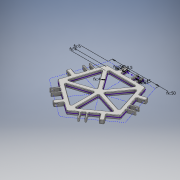
# Autodesk Inventor part: pentagon
Saved by Autodesk Inventor 2016 (Build 200138000, 138)
## iProperties
Created: 2016-11-12
Part Number: pentagon
Material: Generic
Document SubType Name: Modeling
Designer: Chris
Density: 1 g/cm^3
Appearance: Default
Author: Chris
Autodesk Inventor part; units mm, degrees
ref_plane "YZ Plane" through (0, 0, 0) normal (1, 0, 0) x (0, 1, 0)
ref_plane "XZ Plane" through (0, 0, 0) normal (0, 1, 0) x (-1, 0, 0)
ref_plane "XY Plane" through (0, 0, 0) normal (0, 0, 1) x (1, 0, 0)
sketch "Sketch1" plane through (0, 0, 0) normal (0, 0, 1) x (1, 0, 0)
  line L0 (25, 34.409548) -> (40.45085, -13.143278) construction
  line L1 (40.45085, -13.143278) -> (0, -42.53254) construction
  line L2 (0, -42.53254) -> (-40.45085, -13.143278) construction
  line L3 (-40.45085, -13.143278) -> (-25, 34.409548) construction
  line L4 (-25, 34.409548) -> (25, 34.409548) construction
  line L5 (20.640745, 28.409548) -> (33.397427, -10.851482)
  line L6 (33.397427, -10.851482) -> (0, -35.116133)
  line L7 (0, -35.116133) -> (-33.397427, -10.851482)
  line L8 (-33.397427, -10.851482) -> (-20.640745, 28.409548)
  line L9 (-20.640745, 28.409548) -> (20.640745, 28.409548)
  line L10 (0, -35.116133) -> (0, 0) construction
  line L11 (-17.734575, 24.409548) -> (-28.695145, -9.323618)
  line L12 (-28.695145, -9.323618) -> (0, -30.171861)
  line L13 (0, -30.171861) -> (28.695145, -9.323618)
  line L14 (28.695145, -9.323618) -> (17.734575, 24.409548)
  line L15 (17.734575, 24.409548) -> (-17.734575, 24.409548)
  line L16 (-7.5, 34.409548) -> (7.5, 34.409548) construction
  line L17 (4, 34.409548) -> (5.5, 34.409548) construction
  line L18 (5.5, 34.409548) -> (9.5, 34.409548) construction
  line L19 (11, 34.409548) -> (9.5, 34.409548) construction
  line L20 (-9.5, 34.409548) -> (-5.5, 34.409548) construction
  line L21 (-9.5, 28.409548) -> (-5.5, 28.409548)
  line L22 (-5.5, 28.409548) -> (-5.5, 36.409548)
  line L23 (-5.5, 36.409548) -> (-9.5, 36.409548)
  line L24 (-9.5, 36.409548) -> (-9.5, 28.409548)
  line L25 (4, 36.409548) -> (5.5, 36.409548)
  line L26 (5.5, 36.409548) -> (5.5, 28.409548)
  line L27 (5.5, 28.409548) -> (4, 28.409548)
  line L28 (4, 28.409548) -> (4, 36.409548)
  line L29 (9.5, 36.409548) -> (11, 36.409548)
  line L30 (11, 36.409548) -> (11, 28.409548)
  line L31 (11, 28.409548) -> (9.5, 28.409548)
  line L32 (9.5, 28.409548) -> (9.5, 36.409548)
  line L33 (-9.5, 34.409548) -> (-9, 34.409548)
  line L34 (-9.5, 34.409548) -> (-9.5, 35.909548)
  line L35 (-6, 34.409548) -> (-5.5, 34.409548)
  line L36 (-5.5, 34.409548) -> (-5.5, 35.909548)
  arc A0 (-9, 34.409548) -> (-9.5, 35.909548) centre (-11.5, 34.409548) ccw
  arc A1 (-5.5, 35.909548) -> (-6, 34.409548) centre (-3.5, 34.409548) ccw
  line L37 (5.5, 35.909548) -> (5.5, 34.409548)
  line L38 (5.5, 34.409548) -> (6, 34.409548)
  line L39 (9.5, 35.909548) -> (9.5, 34.409548)
  line L40 (9.5, 34.409548) -> (9, 34.409548)
  arc A2 (6, 34.409548) -> (5.5, 35.909548) centre (3.5, 34.409548) ccw
  arc A3 (9.5, 35.909548) -> (9, 34.409548) centre (11.5, 34.409548) ccw
  line L41 (-17.734575, 24.409548) -> (0, 0) construction
  line L42 (-28.695145, -9.323618) -> (0, 0) construction
  line L43 (17.734575, 24.409548) -> (0, 0) construction
  line L44 (28.695145, -9.323618) -> (0, 0) construction
  line L45 (0, 0) -> (-23.21486, 7.542965) construction
  line L46 (0, 24.409548) -> (0, 0) construction
  line L47 (0, 0) -> (23.21486, 7.542965) construction
  line L48 (0, 0) -> (14.347572, -19.747739) construction
  line L49 (-14.347572, -19.747739) -> (0, 0) construction
  line L50 (-18.498507, 22.058407) -> (-3.236068, 1.051462)
  line L51 (-3.236068, 1.051462) -> (-27.931213, -6.972477)
  line L52 (-15.262439, 24.409548) -> (0, 3.402603)
  line L53 (15.262439, 24.409548) -> (0, 3.402603)
  line L54 (18.498507, 22.058407) -> (3.236068, 1.051462)
  line L55 (27.931213, -6.972477) -> (3.236068, 1.051462)
  line L56 (26.695145, -10.776703) -> (2, -2.752764)
  line L57 (2, -2.752764) -> (2, -28.718776)
  line L58 (-2, -28.718776) -> (-2, -2.752764)
  line L59 (-2, -2.752764) -> (-26.695145, -10.776703)
  point P0 (0, 34.409548)
  dimension "d0" = 50
  dimension "d1" = 6
  dimension "d2" = 4
  dimension "d3" = 15
  dimension "d4" = 1.5
  dimension "d5" = 4
  dimension "d6" = 4
  dimension "d9" = 4
  dimension "d12" = 3
  dimension "d13" = 0.5
  dimension "d26" = 4
  constraints: 120 end point, 33 point on line, 16 parallel, 10 equal length, 9 midpoint, 8 horizontal, 8 point on circle, 7 coincident, 6 perpendicular, 5 vertical, 4 centre point, 2 collinear, 2 equal radius, 19 other
  measures "d0" distance of L3.end L0.start
  measures "d1" distance between parallel lines of L9 L4
  measures "d2" distance between parallel lines of L9 L15
  measures "d3" distance of L16.start L16.end
  measures "d4" distance of L19.start L18.end
  measures "d5" distance of L17.end L18.end
  measures "d6" distance of L20.start L20.end
  measures "d9" diameter of L23 L4
  measures "d12" diameter of L34.end L33
  measures "d13" distance of L20.start L33.end
  measures "d26" distance between parallel lines of L52 L50
extrude "Extrusion3" add sketch "Sketch1" along normal mid plane 4 contours L5 L6 L7 L8 L9 | L15 L52 L53 L14 L54 L55 L13 L56 L57 L12 L58 L59 L11 L51 L50
extrude "Extrusion2" add sketch "Sketch1" along normal mid plane 4 contours L9 L32 L29 L30 | L9 L28 L25 L26 | L24 L33 A0 L23 L22 A1 L35 L9 | L24 A0 L33 | L35 A1 L22
revolve "Revolution1" add sketch "Sketch1" angle 360 about axis through (-25, 34.409548, 0) along (1, 0, 0) contours L40 A3 L32 | L26 A2 L38
revolve "Revolution3" cut sketch "Sketch1" angle 360 about axis through (-9.5, 34.409548, 0) along (1, 0, 0) contours L24 A0 L33 | L35 A1 L22
fillet "Fillet5" radius 1 20 edges at (-20.6407, 28.4095, 0) (20.6407, 28.4095, 0) (33.3974, -10.8515, 0) (0, -35.1161, 0) (-33.3974, -10.8515, 0) (-18.4985, 22.0584, 0) (-15.2624, 24.4095, 0) (15.2624, 24.4095, 0) (0, 3.4026, 0) (-3.2361, 1.0515, 0) (-2, -2.7528, 0) (2, -2.7528, 0) (3.2361, 1.0515, 0) (-27.9312, -6.9725, 0) (-26.6951, -10.7767, 0) (-2, -28.7188, 0) (2, -28.7188, 0) (26.6951, -10.7767, 0) (27.9312, -6.9725, 0) (18.4985, 22.0584, 0)
pattern_circular "Circular Pattern1" count 5 over 360 about axis through (0, 0, -10) along (0, 0, 1) of "Extrusion2", "Revolution1", "Revolution3"
fillet "Fillet4" radius 0.75 60 edges at (-30.3002, -22.9903, 0) (-29.0867, -23.872, 0) (-25.8506, -26.2231, 0) (-24.6371, -27.1048, 0) (-16.9514, -32.6888, 0) (-13.7153, -35.0399, 0) (29.0867, -23.872, 0) (25.8506, -26.2231, 0) (18.1649, -31.8071, 0) (16.9514, -32.6888, 0) (13.7153, -35.0399, 0) (12.5018, -35.9216, 0) (38.0267, 0.7895, 0) (37.5632, 2.2161, 0) (36.3271, 6.0204, 0) (35.8636, 7.4469, 0) (32.9279, 16.482, 0) (31.6919, 20.2862, 0) (-9.5, 36.4095, 0) (-5.5, 36.4095, 0) (4, 36.4095, 0) (5.5, 36.4095, 0) (9.5, 36.4095, 0) (11, 36.4095, 0) (-31.6919, 20.2862, 0) (-31.2284, 21.7128, 0) (-32.9279, 16.482, 0) (-33.3915, 15.0554, 0) (-36.3271, 6.0204, 0) (-37.5632, 2.2161, 0) (-9.5, 28.4095, 0) (-5.5, 28.4095, 0) (4, 28.4095, 0) (5.5, 28.4095, 0) (9.5, 28.4095, 0) (11, 28.4095, 0) (24.0834, 17.8141, 0) (25.3195, 14.0098, 0) (28.2552, 4.9748, 0) (28.7187, 3.5482, 0) (29.9547, -0.256, 0) (30.4183, -1.6826, 0) (24.3844, -17.3998, 0) (21.1483, -19.751, 0) (13.4626, -25.3349, 0) (12.2491, -26.2166, 0) (9.0131, -28.5678, 0) (7.7995, -29.4494, 0) (-9.0131, -28.5678, 0) (-12.2491, -26.2166, 0) (-21.1483, -19.751, 0) (-19.9348, -20.6327, 0) (-25.5979, -16.5182, 0) (-24.3844, -17.3998, 0) (-29.9547, -0.256, 0) (-28.7187, 3.5482, 0) (-25.783, 12.5833, 0) (-25.3195, 14.0098, 0) (-24.0834, 17.8141, 0) (-23.6199, 19.2407, 0)
chamfer "Chamfer2" distance 0.4 angle 45 244 edges at (-15.0821, 28.4095, 2) (-20.502, 28.2186, 2) (-22.1267, 23.8363, 2) (-23.7609, 19.5175, 2) (-27.4241, 20.4767, 2) (-31.4151, 20.4272, 2) (-31.0873, 21.436, 2) (-27.8877, 19.0501, 2) (-24.3602, 17.673, 2) (-24.7015, 15.912, 2) (-25.4605, 14.2866, 2) (-29.1237, 15.2459, 2) (-32.7869, 16.2052, 2) (-33.1147, 15.1964, 2) (-29.5872, 13.8193, 2) (-26.0598, 12.4422, 2) (-27.2508, 8.0657, 2) (-28.8597, 3.825, 2) (-32.5229, 4.7843, 2) (-36.1861, 5.7436, 2) (-36.9452, 4.1182, 2) (-37.2864, 2.3572, 2) (-33.759, 0.9801, 2) (-30.2315, -0.397, 2) (-31.6797, -5.5649, 2) (-33.1729, -10.7785, 2) (-29.5072, -13.6779, 2) (-25.9047, -16.5668, 2) (-27.949, -19.7542, 2) (-29.1353, -23.5651, 2) (-29.9933, -22.9417, 2) (-26.7355, -20.6359, 2) (-24.3358, -17.7067, 2) (-22.7663, -18.5754, 2) (-21.4551, -19.7996, 2) (-23.4994, -22.9871, 2) (-24.6857, -26.798, 2) (-25.5438, -26.1745, 2) (-22.2859, -23.8687, 2) (-19.8862, -20.9395, 2) (-16.092, -23.4246, 2) (-12.556, -26.2652, 2) (-14.6003, -29.4527, 2) (-16.6446, -32.6402, 2) (-15.3334, -33.8643, 2) (-13.7639, -34.7331, 2) (-11.3642, -31.8038, 2) (-8.9645, -28.8746, 2) (-4.497, -31.8488, 2) (0, -34.8801, 2) (3.8903, -32.2897, 2) (7.7509, -29.7563, 2) (10.1507, -32.6855, 2) (13.4085, -34.9913, 2) (12.5504, -35.6147, 2) (11.3642, -31.8038, 2) (9.3199, -28.6164, 2) (10.6311, -27.3922, 2) (12.2005, -26.5235, 2) (14.6003, -29.4527, 2) (17.8581, -31.7585, 2) (17, -32.3819, 2) (15.8138, -28.571, 2) (13.7695, -25.3835, 2) (17.3055, -22.543, 2) (21.0997, -20.0578, 2) (23.4994, -22.9871, 2) (25.8992, -25.9163, 2) (27.4686, -25.0476, 2) (28.7798, -23.8234, 2) (26.7355, -20.6359, 2) (24.6912, -17.4484, 2) (28.9004, -14.1188, 2) (33.1729, -10.7785, 2) (31.9115, -6.2782, 2) (30.6951, -1.8236, 2) (34.2225, -0.4465, 2) (37.4222, 1.9393, 2) (37.7499, 0.9306, 2) (33.759, 0.9801, 2) (30.0958, 0.0208, 2) (29.3367, 1.6461, 2) (28.9955, 3.4072, 2) (32.5229, 4.7843, 2) (35.7226, 7.1701, 2) (36.0503, 6.1614, 2) (32.0594, 6.2109, 2) (28.3962, 5.2516, 2) (26.7873, 9.4923, 2) (25.5963, 13.8688, 2) (29.1237, 15.2459, 2) (32.6511, 16.623, 2) (-15.0821, 28.4095, -2) (-9.7197, 28.6292, -2) (-9.5, 32.4095, -2) (-9.2803, 36.1899, -2) (-7.5, 36.4095, -2) (-5.7197, 36.1899, -2) (-5.5, 32.4095, -2) (-5.2803, 28.6292, -2) (-0.75, 28.4095, -2) (3.7803, 28.6292, -2) (4, 32.4095, -2) (4.2197, 36.1899, -2) (5.2803, 36.1899, -2) (5.5, 32.4095, -2) (5.7197, 28.6292, -2) (7.5, 28.4095, -2) (9.2803, 28.6292, -2) (9.5, 32.4095, -2) (9.7197, 36.1899, -2) (10.7803, 36.1899, -2) (11, 32.4095, -2) (11.2197, 28.6292, -2) (15.8321, 28.4095, -2) (20.502, 28.2186, -2) (22.3585, 23.123, -2) (24.2245, 18.0909, -2) (27.8877, 19.0501, -2) (31.5508, 20.0094, -2) (32.3099, 18.3841, -2) (32.6511, 16.623, -2) (29.1237, 15.2459, -2) (25.5963, 13.8688, -2) (26.7873, 9.4923, -2) (28.3962, 5.2516, -2) (32.0594, 6.2109, -2) (35.7226, 7.1701, -2) (36.0503, 6.1614, -2) (32.5229, 4.7843, -2) (28.9955, 3.4072, -2) (29.3367, 1.6461, -2) (30.0958, 0.0208, -2) (33.759, 0.9801, -2) (37.4222, 1.9393, -2) (37.7499, 0.9306, -2) (34.2225, -0.4465, -2) (30.6951, -1.8236, -2) (31.9115, -6.2782, -2) (33.1729, -10.7785, -2) (28.9004, -14.1188, -2) (24.6912, -17.4484, -2) (26.7355, -20.6359, -2) (28.7798, -23.8234, -2) (27.4686, -25.0476, -2) (25.8992, -25.9163, -2) (23.4994, -22.9871, -2) (21.0997, -20.0578, -2) (17.3055, -22.543, -2) (13.7695, -25.3835, -2) (15.8138, -28.571, -2) (17.8581, -31.7585, -2) (17, -32.3819, -2) (14.6003, -29.4527, -2) (12.2005, -26.5235, -2) (10.6311, -27.3922, -2) (9.3199, -28.6164, -2) (11.3642, -31.8038, -2) (13.4085, -34.9913, -2) (12.5504, -35.6147, -2) (10.1507, -32.6855, -2) (7.7509, -29.7563, -2) (3.8903, -32.2897, -2) (0, -34.8801, -2) (-4.497, -31.8488, -2) (-8.9645, -28.8746, -2) (-11.3642, -31.8038, -2) (-13.7639, -34.7331, -2) (-15.3334, -33.8643, -2) (-16.6446, -32.6402, -2) (-14.6003, -29.4527, -2) (-12.556, -26.2652, -2) (-16.092, -23.4246, -2) (-19.8862, -20.9395, -2) (-22.2859, -23.8687, -2) (-24.6857, -26.798, -2) (-25.5438, -26.1745, -2) (-23.4994, -22.9871, -2) (-21.4551, -19.7996, -2) (-22.7663, -18.5754, -2) (-24.3358, -17.7067, -2) (-26.7355, -20.6359, -2) (-29.1353, -23.5651, -2) (-29.9933, -22.9417, -2) (7.4589, 13.6689, -2) (14.1908, 23.8635, -2) (0, 24.4095, -2) (-14.1908, 23.8635, -2) (-7.4589, 13.6689, -2) (0, 4.1039, -2) (7.4589, 13.6689, 2) (0, 4.1039, 2) (-7.4589, 13.6689, 2) (-14.1908, 23.8635, 2) (0, 24.4095, 2) (14.1908, 23.8635, 2) (-3.903, 1.2682, -2) (-15.3049, -2.8699, -2) (-27.0808, -6.122, -2) (-23.2149, 7.543, -2) (-18.3104, 20.8705, -2) (-10.695, 11.3178, -2) (-3.903, 1.2682, 2) (-10.695, 11.3178, 2) (-18.3104, 20.8705, 2) (-23.2149, 7.543, 2) (-27.0808, -6.122, 2) (-15.3049, -2.8699, 2) (-2.4122, -3.3201, -2) (-2, -15.4427, -2) (-2.546, -27.6472, -2) (-14.3476, -19.7477, -2) (-25.5073, -10.9648, -2) (-14.0688, -6.6742, -2) (-2.4122, -3.3201, 2) (-14.0688, -6.6742, 2) (-25.5073, -10.9648, 2) (-14.3476, -19.7477, 2) (-2.546, -27.6472, 2) (-2, -15.4427, 2) (2.4122, -3.3201, -2) (14.0688, -6.6742, -2) (25.5073, -10.9648, -2) (14.3476, -19.7477, -2) (2.546, -27.6472, -2) (2, -15.4427, -2) (2.4122, -3.3201, 2) (2, -15.4427, 2) (2.546, -27.6472, 2) (14.3476, -19.7477, 2) (25.5073, -10.9648, 2) (14.0688, -6.6742, 2) (3.903, 1.2682, -2) (10.695, 11.3178, -2) (18.3104, 20.8705, -2) (23.2149, 7.543, -2) (27.0808, -6.122, -2) (15.3049, -2.8699, -2) (3.903, 1.2682, 2) (15.3049, -2.8699, 2) (27.0808, -6.122, 2) (23.2149, 7.543, 2) (18.3104, 20.8705, 2) (10.695, 11.3178, 2)
equation "\"d0\" = sidelength"
equation "\"d1\" = springlength"
equation "\"d2\" = diam"
equation "\"d3\" = matespace"
equation "\"d4\" = springwidth"
equation "\"d5\" = fingerwidth + 0.5 * tolerance"
equation "\"d6\" = fingerwidth - 0.5 * tolerance"
equation "\"d9\" = diam"
equation "\"d12\" = dentdiam"
equation "\"d13\" = dent"
equation "\"d10\" = diam"
equation "\"sidelength\" = 50"
equation "\"diam\" = 4"
equation "\"dent\" = 0.5"
equation "\"dentdiam\" = 3"
equation "\"tolerance\" = 0"
equation "\"fingerwidth\" = 4"
equation "\"springwidth\" = 1.5"
equation "\"matespace\" = 15"
equation "\"springlength\" = 6"
body "Solid1"
body "Solid2"
